Autodesk Inventor part; units mm, degrees
(part 2 of 2)
  arc A320 (27.3685, 17.399) -> (27.2733, 17.8117) centre (26.4268, 17.3991) ccw
  arc A321 (27.051, 18.0023) -> (27.051, 17.9388) centre (27.051, 17.9706) ccw
  arc A322 (27.2432, 17.8015) -> (27.3033, 17.822) centre (27.2733, 17.8118) ccw
  arc A323 (27.2733, 17.8117) -> (27.051, 17.9705) centre (27.051, 17.7355) ccw
  arc A324 (26.7987, 17.822) -> (26.8588, 17.8015) centre (26.8287, 17.8118) ccw
  arc A325 (27.051, 17.9388) -> (27.051, 18.0023) centre (27.051, 17.9706) ccw
  arc A326 (27.051, 17.9705) -> (26.8288, 17.8117) centre (27.051, 17.7356) ccw
  arc A327 (26.7018, 17.399) -> (26.7653, 17.399) centre (26.7336, 17.399) ccw
  arc A328 (26.8573, 17.7978) -> (26.8002, 17.8257) centre (26.8287, 17.8118) ccw
  arc A329 (26.8288, 17.8117) -> (26.7335, 17.399) centre (27.6752, 17.3989) ccw
  arc A330 (25.5905, 16.8592) -> (25.5905, 16.7958) centre (25.5905, 16.8275) ccw
  arc A331 (26.2255, 16.7958) -> (26.2255, 16.8592) centre (26.2255, 16.8275) ccw
  line L70 (25.5905, 16.8275) -> (26.2255, 16.8275)
  arc A332 (25.9398, 17.9705) -> (25.8763, 17.9705) centre (25.9081, 17.9705) ccw
  arc A333 (25.8763, 16.8275) -> (25.9398, 16.8275) centre (25.9081, 16.8275) ccw
  line L71 (25.908, 17.9705) -> (25.908, 16.8275)
  arc A334 (25.5707, 17.7413) -> (25.6103, 17.6917) centre (25.5905, 17.7165) ccw
  arc A335 (25.9278, 17.9457) -> (25.8882, 17.9953) centre (25.908, 17.9705) ccw
  line L72 (25.5905, 17.7165) -> (25.908, 17.9705)
  arc A336 (3.3655, 16.8592) -> (3.3655, 16.7958) centre (3.3655, 16.8275) ccw
  arc A337 (4.0005, 16.7958) -> (4.0005, 16.8592) centre (4.0005, 16.8275) ccw
  line L73 (3.3655, 16.8275) -> (4.0005, 16.8275)
  arc A338 (3.7148, 17.9705) -> (3.6513, 17.9705) centre (3.683, 17.9705) ccw
  arc A339 (3.6513, 16.8275) -> (3.7148, 16.8275) centre (3.683, 16.8275) ccw
  line L74 (3.683, 17.9705) -> (3.683, 16.8275)
  arc A340 (3.3457, 17.7413) -> (3.3853, 17.6917) centre (3.3655, 17.7165) ccw
  arc A341 (3.7028, 17.9457) -> (3.6632, 17.9953) centre (3.683, 17.9705) ccw
  line L75 (3.3655, 17.7165) -> (3.683, 17.9705)
  arc A342 (23.114, 14.0081) -> (23.114, 13.9319) centre (23.114, 13.97) ccw
  arc A343 (25.146, 13.9319) -> (25.146, 14.0081) centre (25.146, 13.97) ccw
  line L76 (23.114, 13.97) -> (25.146, 13.97)
  arc A344 (25.1191, 13.9969) -> (25.1729, 13.9431) centre (25.146, 13.97) ccw
  arc A345 (25.4269, 14.1971) -> (25.3731, 14.2509) centre (25.4, 14.224) ccw
  line L77 (25.146, 13.97) -> (25.4, 14.224)
  arc A346 (22.5791, 13.9969) -> (22.6329, 13.9431) centre (22.606, 13.97) ccw
  arc A347 (22.8869, 14.1971) -> (22.8331, 14.2509) centre (22.86, 14.224) ccw
  line L78 (22.606, 13.97) -> (22.86, 14.224)
  arc A348 (22.8869, 14.2509) -> (22.8331, 14.1971) centre (22.86, 14.224) ccw
  arc A349 (23.0871, 13.9431) -> (23.1409, 13.9969) centre (23.114, 13.97) ccw
  line L79 (22.86, 14.224) -> (23.114, 13.97)
  arc A350 (25.4269, 14.2509) -> (25.3731, 14.1971) centre (25.4, 14.224) ccw
  arc A351 (25.6271, 13.9431) -> (25.6809, 13.9969) centre (25.654, 13.97) ccw
  line L80 (25.4, 14.224) -> (25.654, 13.97)
  arc A352 (25.3731, 16.2291) -> (25.4269, 16.2829) centre (25.4, 16.256) ccw
  arc A353 (25.1729, 16.5369) -> (25.1191, 16.4831) centre (25.146, 16.51) ccw
  line L81 (25.4, 16.256) -> (25.146, 16.51)
  arc A354 (25.6809, 16.4831) -> (25.6271, 16.5369) centre (25.654, 16.51) ccw
  arc A355 (25.3731, 16.2829) -> (25.4269, 16.2291) centre (25.4, 16.256) ccw
  line L82 (25.654, 16.51) -> (25.4, 16.256)
  arc A356 (27.9019, 13.97) -> (27.9781, 13.97) centre (27.94, 13.97) ccw
  arc A357 (27.9781, 16.51) -> (27.9019, 16.51) centre (27.94, 16.51) ccw
  line L83 (27.94, 13.97) -> (27.94, 16.51)
  arc A358 (27.94, 16.4719) -> (27.94, 16.5481) centre (27.94, 16.51) ccw
  arc A359 (25.654, 16.5481) -> (25.654, 16.4719) centre (25.654, 16.51) ccw
  line L84 (27.94, 16.51) -> (25.654, 16.51)
  arc A360 (25.654, 14.0081) -> (25.654, 13.9319) centre (25.654, 13.97) ccw
  arc A361 (27.94, 13.9319) -> (27.94, 14.0081) centre (27.94, 13.97) ccw
  line L85 (25.654, 13.97) -> (27.94, 13.97)
  arc A362 (25.146, 16.4719) -> (25.146, 16.5481) centre (25.146, 16.51) ccw
  arc A363 (23.114, 16.5481) -> (23.114, 16.4719) centre (23.114, 16.51) ccw
  line L86 (25.146, 16.51) -> (23.114, 16.51)
  arc A364 (22.8331, 16.2291) -> (22.8869, 16.2829) centre (22.86, 16.256) ccw
  arc A365 (22.6329, 16.5369) -> (22.5791, 16.4831) centre (22.606, 16.51) ccw
  line L87 (22.86, 16.256) -> (22.606, 16.51)
  arc A366 (23.1409, 16.4831) -> (23.0871, 16.5369) centre (23.114, 16.51) ccw
  arc A367 (22.8331, 16.2829) -> (22.8869, 16.2291) centre (22.86, 16.256) ccw
  line L88 (23.114, 16.51) -> (22.86, 16.256)
  arc A368 (18.034, 14.0081) -> (18.034, 13.9319) centre (18.034, 13.97) ccw
  arc A369 (20.066, 13.9319) -> (20.066, 14.0081) centre (20.066, 13.97) ccw
  line L89 (18.034, 13.97) -> (20.066, 13.97)
  arc A370 (20.0391, 13.9969) -> (20.0929, 13.9431) centre (20.066, 13.97) ccw
  arc A371 (20.3469, 14.1971) -> (20.2931, 14.2509) centre (20.32, 14.224) ccw
  line L90 (20.066, 13.97) -> (20.32, 14.224)
  arc A372 (20.3469, 14.2509) -> (20.2931, 14.1971) centre (20.32, 14.224) ccw
  arc A373 (20.5471, 13.9431) -> (20.6009, 13.9969) centre (20.574, 13.97) ccw
  line L91 (20.32, 14.224) -> (20.574, 13.97)
  arc A374 (20.066, 16.4719) -> (20.066, 16.5481) centre (20.066, 16.51) ccw
  arc A375 (18.034, 16.5481) -> (18.034, 16.4719) centre (18.034, 16.51) ccw
  line L92 (20.066, 16.51) -> (18.034, 16.51)
  arc A376 (20.6009, 16.4831) -> (20.5471, 16.5369) centre (20.574, 16.51) ccw
  arc A377 (20.2931, 16.2829) -> (20.3469, 16.2291) centre (20.32, 16.256) ccw
  line L93 (20.574, 16.51) -> (20.32, 16.256)
  arc A378 (20.2931, 16.2291) -> (20.3469, 16.2829) centre (20.32, 16.256) ccw
  arc A379 (20.0929, 16.5369) -> (20.0391, 16.4831) centre (20.066, 16.51) ccw
  line L94 (20.32, 16.256) -> (20.066, 16.51)
  arc A380 (20.574, 14.0081) -> (20.574, 13.9319) centre (20.574, 13.97) ccw
  arc A381 (22.606, 13.9319) -> (22.606, 14.0081) centre (22.606, 13.97) ccw
  line L95 (20.574, 13.97) -> (22.606, 13.97)
  arc A382 (22.606, 16.4719) -> (22.606, 16.5481) centre (22.606, 16.51) ccw
  arc A383 (20.574, 16.5481) -> (20.574, 16.4719) centre (20.574, 16.51) ccw
  line L96 (22.606, 16.51) -> (20.574, 16.51)
  arc A384 (14.986, 16.4719) -> (14.986, 16.5481) centre (14.986, 16.51) ccw
  arc A385 (12.954, 16.5481) -> (12.954, 16.4719) centre (12.954, 16.51) ccw
  line L97 (14.986, 16.51) -> (12.954, 16.51)
  arc A386 (15.2131, 16.2291) -> (15.2669, 16.2829) centre (15.24, 16.256) ccw
  arc A387 (15.0129, 16.5369) -> (14.9591, 16.4831) centre (14.986, 16.51) ccw
  line L98 (15.24, 16.256) -> (14.986, 16.51)
  arc A388 (15.5209, 16.4831) -> (15.4671, 16.5369) centre (15.494, 16.51) ccw
  arc A389 (15.2131, 16.2829) -> (15.2669, 16.2291) centre (15.24, 16.256) ccw
  line L99 (15.494, 16.51) -> (15.24, 16.256)
  arc A390 (17.526, 16.4719) -> (17.526, 16.5481) centre (17.526, 16.51) ccw
  arc A391 (15.494, 16.5481) -> (15.494, 16.4719) centre (15.494, 16.51) ccw
  line L100 (17.526, 16.51) -> (15.494, 16.51)
  arc A392 (17.7531, 16.2291) -> (17.8069, 16.2829) centre (17.78, 16.256) ccw
  arc A393 (17.5529, 16.5369) -> (17.4991, 16.4831) centre (17.526, 16.51) ccw
  line L101 (17.78, 16.256) -> (17.526, 16.51)
  arc A394 (18.0609, 16.4831) -> (18.0071, 16.5369) centre (18.034, 16.51) ccw
  arc A395 (17.7531, 16.2829) -> (17.8069, 16.2291) centre (17.78, 16.256) ccw
  line L102 (18.034, 16.51) -> (17.78, 16.256)
  arc A396 (17.8069, 14.2509) -> (17.7531, 14.1971) centre (17.78, 14.224) ccw
  arc A397 (18.0071, 13.9431) -> (18.0609, 13.9969) centre (18.034, 13.97) ccw
  line L103 (17.78, 14.224) -> (18.034, 13.97)
  arc A398 (17.4991, 13.9969) -> (17.5529, 13.9431) centre (17.526, 13.97) ccw
  arc A399 (17.8069, 14.1971) -> (17.7531, 14.2509) centre (17.78, 14.224) ccw
  line L104 (17.526, 13.97) -> (17.78, 14.224)
  arc A400 (15.494, 14.0081) -> (15.494, 13.9319) centre (15.494, 13.97) ccw
  arc A401 (17.526, 13.9319) -> (17.526, 14.0081) centre (17.526, 13.97) ccw
  line L105 (15.494, 13.97) -> (17.526, 13.97)
  arc A402 (15.2669, 14.2509) -> (15.2131, 14.1971) centre (15.24, 14.224) ccw
  arc A403 (15.4671, 13.9431) -> (15.5209, 13.9969) centre (15.494, 13.97) ccw
  line L106 (15.24, 14.224) -> (15.494, 13.97)
  arc A404 (76.2324, 34.6527) -> (76.2324, 35.1748) centre (76.2324, 34.9138) ccw
  arc A405 (14.9591, 13.9969) -> (15.0129, 13.9431) centre (14.986, 13.97) ccw
  arc A406 (15.2669, 14.1971) -> (15.2131, 14.2509) centre (15.24, 14.224) ccw
  line L107 (14.986, 13.97) -> (15.24, 14.224)
  arc A407 (12.954, 14.0081) -> (12.954, 13.9319) centre (12.954, 13.97) ccw
  arc A408 (14.986, 13.9319) -> (14.986, 14.0081) centre (14.986, 13.97) ccw
  line L108 (12.954, 13.97) -> (14.986, 13.97)
  arc A409 (4.826, 16.4719) -> (4.826, 16.5481) centre (4.826, 16.51) ccw
  arc A410 (2.54, 16.5481) -> (2.54, 16.4719) centre (2.54, 16.51) ccw
  line L109 (4.826, 16.51) -> (2.54, 16.51)
  arc A411 (5.0531, 16.2291) -> (5.1069, 16.2829) centre (5.08, 16.256) ccw
  arc A412 (4.8529, 16.5369) -> (4.7991, 16.4831) centre (4.826, 16.51) ccw
  line L110 (5.08, 16.256) -> (4.826, 16.51)
  arc A413 (5.3609, 16.4831) -> (5.3071, 16.5369) centre (5.334, 16.51) ccw
  arc A414 (5.0531, 16.2829) -> (5.1069, 16.2291) centre (5.08, 16.256) ccw
  line L111 (5.334, 16.51) -> (5.08, 16.256)
  arc A415 (7.366, 16.4719) -> (7.366, 16.5481) centre (7.366, 16.51) ccw
  arc A416 (5.334, 16.5481) -> (5.334, 16.4719) centre (5.334, 16.51) ccw
  line L112 (7.366, 16.51) -> (5.334, 16.51)
  arc A417 (7.5931, 16.2291) -> (7.6469, 16.2829) centre (7.62, 16.256) ccw
  arc A418 (7.3929, 16.5369) -> (7.3391, 16.4831) centre (7.366, 16.51) ccw
  line L113 (7.62, 16.256) -> (7.366, 16.51)
  arc A419 (7.9009, 16.4831) -> (7.8471, 16.5369) centre (7.874, 16.51) ccw
  arc A420 (7.5931, 16.2829) -> (7.6469, 16.2291) centre (7.62, 16.256) ccw
  line L114 (7.874, 16.51) -> (7.62, 16.256)
  arc A421 (9.906, 16.4719) -> (9.906, 16.5481) centre (9.906, 16.51) ccw
  arc A422 (7.874, 16.5481) -> (7.874, 16.4719) centre (7.874, 16.51) ccw
  line L115 (9.906, 16.51) -> (7.874, 16.51)
  arc A423 (10.1331, 16.2291) -> (10.1869, 16.2829) centre (10.16, 16.256) ccw
  arc A424 (9.9329, 16.5369) -> (9.8791, 16.4831) centre (9.906, 16.51) ccw
  line L116 (10.16, 16.256) -> (9.906, 16.51)
  arc A425 (10.4409, 16.4831) -> (10.3871, 16.5369) centre (10.414, 16.51) ccw
  arc A426 (10.1331, 16.2829) -> (10.1869, 16.2291) centre (10.16, 16.256) ccw
  line L117 (10.414, 16.51) -> (10.16, 16.256)
  arc A427 (12.446, 16.4719) -> (12.446, 16.5481) centre (12.446, 16.51) ccw
  arc A428 (10.414, 16.5481) -> (10.414, 16.4719) centre (10.414, 16.51) ccw
  line L118 (12.446, 16.51) -> (10.414, 16.51)
  arc A429 (12.6731, 16.2291) -> (12.7269, 16.2829) centre (12.7, 16.256) ccw
  arc A430 (12.4729, 16.5369) -> (12.4191, 16.4831) centre (12.446, 16.51) ccw
  line L119 (12.7, 16.256) -> (12.446, 16.51)
  arc A431 (12.9809, 16.4831) -> (12.9271, 16.5369) centre (12.954, 16.51) ccw
  arc A432 (12.6731, 16.2829) -> (12.7269, 16.2291) centre (12.7, 16.256) ccw
  line L120 (12.954, 16.51) -> (12.7, 16.256)
  arc A433 (12.7269, 14.2509) -> (12.6731, 14.1971) centre (12.7, 14.224) ccw
  arc A434 (12.9271, 13.9431) -> (12.9809, 13.9969) centre (12.954, 13.97) ccw
  line L121 (12.7, 14.224) -> (12.954, 13.97)
  arc A435 (12.4191, 13.9969) -> (12.4729, 13.9431) centre (12.446, 13.97) ccw
  arc A436 (12.7269, 14.1971) -> (12.6731, 14.2509) centre (12.7, 14.224) ccw
  line L122 (12.446, 13.97) -> (12.7, 14.224)
  arc A437 (10.414, 14.0081) -> (10.414, 13.9319) centre (10.414, 13.97) ccw
  arc A438 (12.446, 13.9319) -> (12.446, 14.0081) centre (12.446, 13.97) ccw
  line L123 (10.414, 13.97) -> (12.446, 13.97)
  arc A439 (10.1869, 14.2509) -> (10.1331, 14.1971) centre (10.16, 14.224) ccw
  arc A440 (10.3871, 13.9431) -> (10.4409, 13.9969) centre (10.414, 13.97) ccw
  line L124 (10.16, 14.224) -> (10.414, 13.97)
  arc A441 (9.8791, 13.9969) -> (9.9329, 13.9431) centre (9.906, 13.97) ccw
  arc A442 (10.1869, 14.1971) -> (10.1331, 14.2509) centre (10.16, 14.224) ccw
  line L125 (9.906, 13.97) -> (10.16, 14.224)
  arc A443 (7.874, 14.0081) -> (7.874, 13.9319) centre (7.874, 13.97) ccw
  arc A444 (9.906, 13.9319) -> (9.906, 14.0081) centre (9.906, 13.97) ccw
  line L126 (7.874, 13.97) -> (9.906, 13.97)
  arc A445 (7.6469, 14.2509) -> (7.5931, 14.1971) centre (7.62, 14.224) ccw
  arc A446 (7.8471, 13.9431) -> (7.9009, 13.9969) centre (7.874, 13.97) ccw
  line L127 (7.62, 14.224) -> (7.874, 13.97)
  arc A447 (7.3391, 13.9969) -> (7.3929, 13.9431) centre (7.366, 13.97) ccw
  arc A448 (7.6469, 14.1971) -> (7.5931, 14.2509) centre (7.62, 14.224) ccw
  line L128 (7.366, 13.97) -> (7.62, 14.224)
  arc A449 (5.334, 14.0081) -> (5.334, 13.9319) centre (5.334, 13.97) ccw
  arc A450 (7.366, 13.9319) -> (7.366, 14.0081) centre (7.366, 13.97) ccw
  line L129 (5.334, 13.97) -> (7.366, 13.97)
  arc A451 (5.1069, 14.2509) -> (5.0531, 14.1971) centre (5.08, 14.224) ccw
  arc A452 (5.3071, 13.9431) -> (5.3609, 13.9969) centre (5.334, 13.97) ccw
  line L130 (5.08, 14.224) -> (5.334, 13.97)
  arc A453 (4.7991, 13.9969) -> (4.8529, 13.9431) centre (4.826, 13.97) ccw
  arc A454 (5.1069, 14.1971) -> (5.0531, 14.2509) centre (5.08, 14.224) ccw
  line L131 (4.826, 13.97) -> (5.08, 14.224)
  arc A455 (2.54, 14.0081) -> (2.54, 13.9319) centre (2.54, 13.97) ccw
  arc A456 (4.826, 13.9319) -> (4.826, 14.0081) centre (4.826, 13.97) ccw
  line L132 (2.54, 13.97) -> (4.826, 13.97)
  arc A457 (2.5781, 16.51) -> (2.5019, 16.51) centre (2.54, 16.51) ccw
  arc A458 (2.5019, 13.97) -> (2.5781, 13.97) centre (2.54, 13.97) ccw
  line L133 (2.54, 16.51) -> (2.54, 13.97)
  arc A459 (26.4854, 3.5459) -> (26.587, 3.5459) centre (26.5362, 3.5459) ccw
  arc A460 (26.587, 10.0959) -> (26.4854, 10.0959) centre (26.5362, 10.0959) ccw
  line L134 (26.5362, 3.5459) -> (26.5362, 10.0959)
  arc A461 (33.5282, 3.4951) -> (33.5282, 3.5967) centre (33.5282, 3.5459) ccw
  arc A462 (26.5362, 3.5967) -> (26.5362, 3.4951) centre (26.5362, 3.5459) ccw
  line L135 (33.5282, 3.5459) -> (26.5362, 3.5459)
  arc A463 (44.2862, 3.4951) -> (44.2862, 3.5967) centre (44.2862, 3.5459) ccw
  arc A464 (37.2942, 3.5967) -> (37.2942, 3.4951) centre (37.2942, 3.5459) ccw
  line L136 (44.2862, 3.5459) -> (37.2942, 3.5459)
  arc A465 (44.337, 10.0959) -> (44.2354, 10.0959) centre (44.2862, 10.0959) ccw
  arc A466 (44.2354, 3.5459) -> (44.337, 3.5459) centre (44.2862, 3.5459) ccw
  line L137 (44.2862, 10.0959) -> (44.2862, 3.5459)
  arc A467 (26.5362, 10.1467) -> (26.5362, 10.0451) centre (26.5362, 10.0959) ccw
  arc A468 (44.2862, 10.0451) -> (44.2862, 10.1467) centre (44.2862, 10.0959) ccw
  line L138 (26.5362, 10.0959) -> (44.2862, 10.0959)
  arc A469 (25.3604, 2.6209) -> (25.462, 2.6209) centre (25.4112, 2.6209) ccw
  arc A470 (25.462, 11.0209) -> (25.3604, 11.0209) centre (25.4112, 11.0209) ccw
  line L139 (25.4112, 2.6209) -> (25.4112, 11.0209)
  arc A471 (33.5282, 2.5701) -> (33.5282, 2.6717) centre (33.5282, 2.6209) ccw
  arc A472 (25.4112, 2.6717) -> (25.4112, 2.5701) centre (25.4112, 2.6209) ccw
  line L140 (33.5282, 2.6209) -> (25.4112, 2.6209)
  arc A473 (37.2942, 2.5701) -> (37.2942, 2.6717) centre (37.2942, 2.6209) ccw
  arc A474 (33.5282, 2.6717) -> (33.5282, 2.5701) centre (33.5282, 2.6209) ccw
  line L141 (37.2942, 2.6209) -> (33.5282, 2.6209)
  arc A475 (33.579, 4.1709) -> (33.4774, 4.1709) centre (33.5282, 4.1709) ccw
  arc A476 (33.4774, 2.6209) -> (33.579, 2.6209) centre (33.5282, 2.6209) ccw
  line L142 (33.5282, 4.1709) -> (33.5282, 2.6209)
  arc A477 (37.2942, 4.1201) -> (37.2942, 4.2217) centre (37.2942, 4.1709) ccw
  arc A478 (33.5282, 4.2217) -> (33.5282, 4.1201) centre (33.5282, 4.1709) ccw
  line L143 (37.2942, 4.1709) -> (33.5282, 4.1709)
  arc A479 (37.2434, 2.6209) -> (37.345, 2.6209) centre (37.2942, 2.6209) ccw
  arc A480 (37.345, 4.1709) -> (37.2434, 4.1709) centre (37.2942, 4.1709) ccw
  line L144 (37.2942, 2.6209) -> (37.2942, 4.1709)
  arc A481 (39.8702, 2.5701) -> (39.8702, 2.6717) centre (39.8702, 2.6209) ccw
  arc A482 (37.2942, 2.6717) -> (37.2942, 2.5701) centre (37.2942, 2.6209) ccw
  line L145 (39.8702, 2.6209) -> (37.2942, 2.6209)
  arc A483 (39.921, 2.9209) -> (39.8194, 2.9209) centre (39.8702, 2.9209) ccw
  arc A484 (39.8194, 2.6209) -> (39.921, 2.6209) centre (39.8702, 2.6209) ccw
  line L146 (39.8702, 2.9209) -> (39.8702, 2.6209)
  arc A485 (41.3492, 2.8701) -> (41.3492, 2.9717) centre (41.3492, 2.9209) ccw
  arc A486 (39.8702, 2.9717) -> (39.8702, 2.8701) centre (39.8702, 2.9209) ccw
  line L147 (41.3492, 2.9209) -> (39.8702, 2.9209)
  arc A487 (41.2984, 2.6209) -> (41.4, 2.6209) centre (41.3492, 2.6209) ccw
  arc A488 (41.4, 2.9209) -> (41.2984, 2.9209) centre (41.3492, 2.9209) ccw
  line L148 (41.3492, 2.6209) -> (41.3492, 2.9209)
  arc A489 (45.4112, 2.5701) -> (45.4112, 2.6717) centre (45.4112, 2.6209) ccw
  arc A490 (41.3492, 2.6717) -> (41.3492, 2.5701) centre (41.3492, 2.6209) ccw
  line L149 (45.4112, 2.6209) -> (41.3492, 2.6209)
  arc A491 (45.462, 11.0209) -> (45.3604, 11.0209) centre (45.4112, 11.0209) ccw
  arc A492 (45.3604, 2.6209) -> (45.462, 2.6209) centre (45.4112, 2.6209) ccw
  line L150 (45.4112, 11.0209) -> (45.4112, 2.6209)
  arc A493 (25.4112, 11.0717) -> (25.4112, 10.9701) centre (25.4112, 11.0209) ccw
  arc A494 (45.4112, 10.9701) -> (45.4112, 11.0717) centre (45.4112, 11.0209) ccw
  line L151 (25.4112, 11.0209) -> (45.4112, 11.0209)
  arc A495 (3.6673, 3.5601) -> (3.7689, 3.5601) centre (3.7181, 3.5601) ccw
  arc A496 (3.7689, 10.1101) -> (3.6673, 10.1101) centre (3.7181, 10.1101) ccw
  line L152 (3.7181, 3.5601) -> (3.7181, 10.1101)
  arc A497 (10.7101, 3.5093) -> (10.7101, 3.6109) centre (10.7101, 3.5601) ccw
  arc A498 (3.7181, 3.6109) -> (3.7181, 3.5093) centre (3.7181, 3.5601) ccw
  line L153 (10.7101, 3.5601) -> (3.7181, 3.5601)
  arc A499 (21.4681, 3.5093) -> (21.4681, 3.6109) centre (21.4681, 3.5601) ccw
  arc A500 (14.4761, 3.6109) -> (14.4761, 3.5093) centre (14.4761, 3.5601) ccw
  line L154 (21.4681, 3.5601) -> (14.4761, 3.5601)
  arc A501 (21.5189, 10.1101) -> (21.4173, 10.1101) centre (21.4681, 10.1101) ccw
  arc A502 (21.4173, 3.5601) -> (21.5189, 3.5601) centre (21.4681, 3.5601) ccw
  line L155 (21.4681, 10.1101) -> (21.4681, 3.5601)
  arc A503 (3.7181, 10.1609) -> (3.7181, 10.0593) centre (3.7181, 10.1101) ccw
  arc A504 (21.4681, 10.0593) -> (21.4681, 10.1609) centre (21.4681, 10.1101) ccw
  line L156 (3.7181, 10.1101) -> (21.4681, 10.1101)
  arc A505 (2.5423, 2.6351) -> (2.6439, 2.6351) centre (2.5931, 2.6351) ccw
  constraints: 1131 point on circle, 506 centre point, 314 end point, 155 point on line, 14 midpoint
sketch "Sketch8" plane through (0, 0, 0) normal (0, 0, 1) x (1, 0, 0)
  line L0 (0, 0) -> (106.66, 0)
  line L1 (106.66, 0) -> (106.66, 46.91) construction
  line L2 (106.66, 46.91) -> (0, 46.91)
  line L3 (0, 46.91) -> (0, 0) construction
  circle A0 centre (102.615, 42.9184) radius 1.51 projected
  circle A1 centre (102.502, 4.0549) radius 1.51 projected
  circle A2 centre (37.3779, 20.3594) radius 1.51 projected
  circle A3 centre (6.998, 20.3594) radius 1.51 projected
  arc A4 (12.1633, 26.1146) -> (12.1633, 45.1146) centre (12.1633, 35.6146) ccw projected
  arc A5 (12.1633, 45.1146) -> (12.1633, 26.1146) centre (12.1633, 35.6146) ccw projected
  arc A6 (33.6686, 45.1146) -> (33.6686, 26.1146) centre (33.6686, 35.6146) ccw projected
  arc A7 (33.6686, 26.1146) -> (33.6686, 45.1146) centre (33.6686, 35.6146) ccw projected
  arc A8 (55.174, 45.1146) -> (55.174, 26.1146) centre (55.174, 35.6146) ccw projected
  arc A9 (55.174, 26.1146) -> (55.174, 45.1146) centre (55.174, 35.6146) ccw projected
  arc A10 (76.9333, 45.1146) -> (76.9333, 26.1146) centre (76.9333, 35.6146) ccw projected
  arc A11 (76.9333, 26.1146) -> (76.9333, 45.1146) centre (76.9333, 35.6146) ccw projected
  arc A12 (57.7921, 21.5907) -> (57.7921, 2.5907) centre (57.7921, 12.0907) ccw projected
  arc A13 (57.7921, 2.5907) -> (57.7921, 21.5907) centre (57.7921, 12.0907) ccw projected
  arc A14 (78.1431, 21.5907) -> (78.1431, 2.5907) centre (78.1431, 12.0907) ccw projected
  arc A15 (78.1431, 2.5907) -> (78.1431, 21.5907) centre (78.1431, 12.0907) ccw projected
  arc A16 (95.25, 33.63) -> (95.25, 14.63) centre (95.25, 24.13) ccw projected
  arc A17 (95.25, 14.63) -> (95.25, 33.63) centre (95.25, 24.13) ccw projected
  line L4 (-1.915, 46.91) -> (108.575, 46.91)
  line L5 (108.575, 46.91) -> (108.575, 0)
  line L6 (108.575, 0) -> (-1.915, 0)
  line L7 (-1.915, 0) -> (-1.915, 46.91)
  line L8 (108.575, 0) -> (-1.915, 46.91) construction
  line L9 (109.575, -1) -> (-2.915, -1)
  line L10 (-2.915, -1) -> (-2.915, 47.91)
  line L11 (-2.915, 47.91) -> (109.575, 47.91)
  line L12 (109.575, 47.91) -> (109.575, -1)
  line L13 (109.575, -1) -> (-2.915, 47.91) construction
  line L14 (-2.915, -1) -> (109.575, 47.91) construction
  point P0 (53.33, 23.455)
  dimension "d0" = 106.66
  dimension "d1" = 46.91
  dimension "d4" = 1.915
  dimension "d5" = 1.915
  dimension "d6" = 1
  dimension "d7" = 1
  constraints: 30 end point, 6 parallel, 3 horizontal, 3 midpoint, 3 perpendicular, 2 collinear
  measures "d0" distance of L2.end L1.end
  measures "d1" distance of L0.end L1.end
  measures "d4" distance between parallel lines of L3 L7
  measures "d5" distance between parallel lines of L5 L1
  measures "d6" distance between parallel lines of L11 L2
  measures "d7" distance between parallel lines of L10 L7
extrude "Extrusion1" add sketch "Sketch8" along normal blind 3 contours L6 L7 L4 L2 L5 L0 | L9 L10 L11 L12
body "Solid1"
